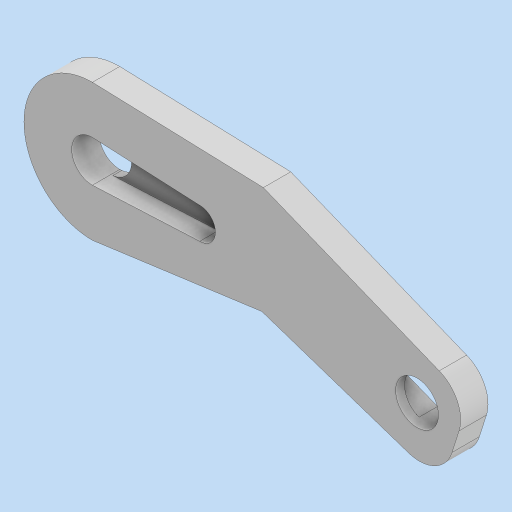
# Autodesk Inventor part: pata_superior_v3
Saved by Autodesk Inventor 2024 (Build 280153000, 153)
## iProperties
Created: 2024-07-27
Part Number: pata_superior_v3
Material: Generic
Document SubType Name: Modeling
Designer: MxMon
Density: 1 g/cm^3
Appearance: Default
Author: MxMon
Autodesk Inventor part; units mm, degrees
ref_plane "YZ Plane" through (0, 0, 0) normal (1, 0, 0) x (0, 1, 0)
ref_plane "XZ Plane" through (0, 0, 0) normal (0, 1, 0) x (-1, 0, 0)
ref_plane "XY Plane" through (0, 0, 0) normal (0, 0, 1) x (1, 0, 0)
sketch "Sketch1" plane through (0, 0, 0) normal (0, 0, 1) x (1, 0, 0)
  arc A0 (0.2884, 3.0112) -> (0.2884, -3.0112) centre (0, 0) ccw
  arc A1 (15.7, -2.275) -> (15.7, 2.275) centre (15.7, 0) ccw
  line L0 (0, 3.025) -> (15.7, 2.275)
  line L1 (0, -3.025) -> (15.7, -2.275)
  dimension "d0" = 6.05
  dimension "d2" = 15.7
  dimension "d3" = 4.55
  constraints: 6 point on circle, 4 end point, 4 vertical alignment, 2 centre point, 2 point on line, 1 coincident, 1 horizontal alignment
  measures "d0" diameter of A0
  measures "d2" distance of A1.centre point (0, 0)
  measures "d3" distance of L1.end L0.end
extrude "Extrusion1" add sketch "Sketch1" along normal blind 4 contours L0 A1 L1 A0
sketch "Sketch6" plane through (0, 0, 4) normal (0, 0, 1) x (1, 0, 0)
  arc A0 (0.6699, 9.9775) -> (2.6736, -9.636) centre (0, 0) ccw
  line L0 (0, 10) -> (24.986, 9.1622)
  line L1 (0, -10) -> (24.7714, -6.6271)
  line L2 (24.986, 9.1622) -> (54.986, -2.9102)
  line L3 (24.7714, -6.6271) -> (51.0332, -15.4223)
  line L4 (54.986, -2.9102) -> (51.0332, -15.4223)
  line L5 (15.7, 2.275) -> (0, 3.025) projected
  arc A1 (0, 3.025) -> (0, -3.025) centre (0, 0) ccw projected
  line L6 (0, -3.025) -> (15.7, -2.275) projected
  arc A2 (15.7, -2.275) -> (15.7, 2.275) centre (15.7, 0) ccw projected
  dimension "d32" = 20
  dimension "d33" = 25
  dimension "d34" = 25
  dimension "d37" = 160
  dimension "d39" = 30
  dimension "d56" = 51.0332
  dimension "d82" = 9.674
  dimension "d83" = 13.1217
  dimension "d84" = 153.73
  constraints: 10 end point, 4 point on circle, 2 point on line, 2 vertical alignment, 1 centre point, 1 coincident
  measures "d32" diameter of A0
  measures "d33" distance of L0.start L0.end
  measures "d34" distance of L1.start L1.end
  measures "d37" angle of L2 L0
  measures "d39" horizontal distance of L0.end L2.end
  measures "d56" horizontal distance of L3.end L1.start
  measures "d82" angle of L1 L0
  measures "d83" distance of L2.end L3.end
  measures "d84" angle of L3 L1
extrude "Extrusion5" add sketch "Sketch6" against normal blind 4 contours L0 L2 L4 L3 L1 A0
sketch "Sketch8" plane through (0, 0, 4) normal (0, 0, 1) x (1, 0, 0)
  line L0 (0, -3.025) -> (15.7, -2.275) projected
  arc A0 (0.2884, 3.0112) -> (0.2884, -3.0112) centre (0, 0) ccw projected
  line L1 (0, 3.025) -> (15.7, 2.275) projected
  arc A1 (15.7, -2.275) -> (15.7, 2.275) centre (15.7, 0) ccw projected
extrude "Extrusion8" cut sketch "Sketch8" against normal blind 2.7 contours A0 L1 A1 L0
sketch "Sketch9" plane through (0, 0, 1.3) normal (0, 0, 1) x (1, 0, 0)
  line L0 (15.7, -2.275) -> (0, -3.025) projected
  circle A0 centre (0, 0) radius 3.025
  point P0 (0.2884, -3.0112)
  constraints: 1 coincident, 3 other
extrude "Extrusion9" cut sketch "Sketch9" against normal through all
sketch "Sketch11" plane through (0, 0, 0) normal (0, 0, -1) x (-1, 0, 0)
  arc A0 (-48.1186, -3.7877) -> (-46.1454, -9.6796) centre (-47.4519, -6.8408) ccw
  arc A1 (-31.8422, -4.0122) -> (-33.2871, 0.3023) centre (-32.5646, -1.855) ccw
  line L0 (-53.146, -8.7478) -> (-23.9305, 1.0366) construction
  line L1 (-48.4443, -3.8776) -> (-33.2871, 0.3023)
  line L2 (-46.4595, -9.804) -> (-31.8422, -4.0122)
  line L3 (-54.986, -2.9102) -> (-51.0332, -15.4223) projected
  line L4 (-51.0332, -15.4223) -> (-24.7714, -6.6271) projected
  point P0 (0, 0)
  dimension "d60" = 6.25
  dimension "d64" = 4.55
  dimension "d65" = 3.125
  dimension "d66" = 2.275
  dimension "d74" = 6
  dimension "d75" = 7
  dimension "d77" = 15.7
  constraints: 6 end point, 5 point on circle, 4 point on line, 2 centre point, 2 symmetric about line, 1 parallel
  measures "d60" diameter of A0
  measures "d64" diameter of A1
  measures "d65" distance from line of L0 L1.start
  measures "d66" distance from line of L1.end L0
  measures "d74" distance from line of L3 A0.centre
  measures "d75" distance from line of L4 A0.centre
  measures "d77" distance of A1.centre A0.centre
fillet "Fillet3" radius 5 2 edges at (54.986, -2.9102, 2) (51.0332, -15.4223, 2)
extrude "Extrusion12" cut sketch "Sketch11" against normal blind 2.7 contours L1 A1 L2 A0
sketch "Sketch14" plane through (0, 0, 2.7) normal (0, 0, -1) x (-1, 0, 0)
  arc A0 (-48.4443, -3.8776) -> (-46.4595, -9.804) centre (-47.4519, -6.8408) ccw projected
  circle A1 centre (-47.4519, -6.8408) radius 3.125
  point P0 (0, 0)
  point P1 (-48.4443, -3.8776)
  constraints: 1 coincident, 3 other
extrude "Extrusion13" cut sketch "Sketch14" against normal blind 2.7
body "Solid1"
